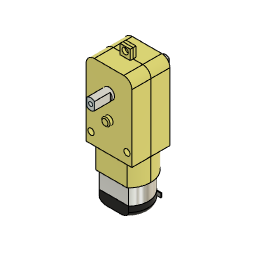
DC 3777 v3 (Autodesk Fusion 360 design; units mm, degrees)
Autodesk Fusion 360 part; units mm, degrees
sketch "main" plane through (0, 0, 0) normal (0, 1, 0) x (1, 0, 0)
  circle A0 centre (0, 0) radius 2.7
  line L0 (-11.2, -11.2) -> (11.2, -11.2)
  line L1 (11.2, -11.2) -> (11.2, 51)
  line L2 (11.2, 51) -> (-11.2, 51)
  line L3 (-11.2, 51) -> (-11.2, -11.2)
  line L4 (0, -11.2) -> (0, 51) construction
  line L5 (-2.5, -16) -> (2.5, -16)
  line L6 (2.5, -16) -> (2.5, -11.2)
  line L7 (2.5, -11.2) -> (-2.5, -11.2)
  line L8 (-2.5, -11.2) -> (-2.5, -16)
  circle A1 centre (0, -14) radius 1.5
  line L9 (-11.2, 25.8) -> (11.2, 25.8)
  line L10 (-1.85, 2.7) -> (1.85, 2.7)
  line L11 (1.85, 2.7) -> (1.85, -2.7)
  line L12 (1.85, -2.7) -> (-1.85, -2.7)
  line L13 (-1.85, -2.7) -> (-1.85, 2.7)
  line L14 (-1.85, 2.7) -> (1.85, -2.7) construction
  line L15 (1.85, 2.7) -> (-1.85, -2.7) construction
  circle A2 centre (8.8, 20.6) radius 1.5
  circle A3 centre (-8.8, 20.6) radius 1.5
  line L16 (8.8, 20.6) -> (-8.8, 20.6) construction
  circle A4 centre (0, 0) radius 0.975
  dimension "d1" = 5.4
  dimension "d2" = 22.4
  dimension "d3" = 62.2
  dimension "d4" = 11.2
  dimension "d5" = 5
  dimension "d7" = 3
  dimension "d8" = 2
  dimension "d10" = 3.7
  dimension "d11" = 5.4
  dimension "d21" = 3
  dimension "d22" = 8.8
  dimension "d23" = 3
  dimension "d24" = 8.8
  dimension "d25" = 31.8
  dimension "d52" = 37
  dimension "d61" = 1.95
  dimension "d62" = 4.8
  constraint coincident A0.centre A4.centre
  constraint horizontal L0
  constraint vertical L1
  constraint horizontal L2
  constraint vertical L3
  constraint midpoint L0 L4.start
  constraint midpoint L2 L4.end
  constraint coincident A0.centre L4
  constraint horizontal L5
  constraint vertical L6
  constraint horizontal L7
  constraint vertical L8
  constraint midpoint L0 L7
  constraint coincident L3 L9.start
  constraint coincident L1 L9.end
  constraint perpendicular L1 L9
  constraint perpendicular L10 L11
  constraint parallel L10 L12
  constraint parallel L11 L13
  constraint horizontal L10
  constraint coincident L14 A0.centre
  constraint coincident L15 A0.centre
  constraint coincident A2.centre L16.start
  constraint coincident A3.centre L16.end
  constraint horizontal L16
  measures "d1" diameter of A0
  measures "d2" distance of L0.start L0.end
  measures "d3" distance of L0.end L1.end
  measures "d4" distance of A0.centre L0
  measures "d5" distance of L5.start L5.end
  measures "d7" diameter of A1
  measures "d8" distance of L5 A1.centre
  measures "d10" distance of L11.end L12.end
  measures "d11" distance of L10.end L11.end
  measures "d21" diameter of A2
  measures "d22" distance of L4 A2.centre
  measures "d23" diameter of A3
  measures "d24" distance of L4 A3.centre
  measures "d25" distance of L0 A2.centre
  measures "d52" distance of L0 L9
  measures "d61" diameter of A4
  measures "d62" distance of L5.end L6.end
extrude "Extrude1" add sketch "main" along normal mid plane 18.6 contours A0 L10 L11 | A0 L11 L12 | A0 L10 L13 | A0 L12 L13 | L0 L1 L3 L7 L9 makes body 1
extrude "Extrude2" add sketch "main" along normal mid plane 2.8 contours L0 L5 L6 L7 L8 bodies 1
extrude "Extrude3" add sketch "main" along normal mid plane 21 separate body contours A0 L11 | A0 L11 L13 | A0 L13 | A4 makes body 2
extrude "Extrude4" add sketch "main" along normal mid plane 36.6 contours A0 L11 L13 bodies 2
fillet "Fillet1" radius 4 2 edges at (11.2, 0, 11.2) (-11.2, 0, 11.2) on bodies 1
sketch "bottom" plane through (0, 0, -25.8) normal (0, 0, -1) x (1, 0, 0)
  line L0 (-11.2, 9.3) -> (-11.2, -9.3)
  line L1 (-11.2, -9.3) -> (11.2, -9.3)
  line L2 (11.2, -9.3) -> (11.2, 9.3)
  line L3 (11.2, 9.3) -> (-11.2, 9.3)
  circle A0 centre (0, 0) radius 11.15
  line L4 (-11.2, 8.1) -> (11.2, 8.1)
  dimension "d26" = 22.3
  dimension "d29" = 1.2
  constraint coincident A0.centre origin
  constraint coincident L0 L4.start
  constraint coincident L2 L4.end
  constraint horizontal L4
  measures "d26" diameter of A0
  measures "d29" distance of L3 L4
extrude "Extrude5" add sketch "bottom" along normal blind 11 contours L1 A0 L4 bodies 1
sketch "more" plane through (0, 0, -36.8) normal (0, 0, -1) x (1, 0, 0)
  arc A0 (-7.6624, 8.1) -> (-6.1508, -9.3) centre (0, 0) ccw
  line L0 (-6.1508, -9.3) -> (6.1508, -9.3)
  arc A1 (6.1508, -9.3) -> (7.6624, 8.1) centre (0, 0) ccw
  line L1 (7.6624, 8.1) -> (-7.6624, 8.1)
  circle A2 centre (0, 0) radius 4.95
  arc A3 (-7.1689, 6.9) -> (-5.7786, -8.1) centre (0, 0) ccw
  line L2 (-5.7786, -8.1) -> (5.7786, -8.1)
  arc A4 (5.7786, -8.1) -> (7.1689, 6.9) centre (0, 0) ccw
  line L3 (7.1689, 6.9) -> (-7.1689, 6.9)
  line L4 (-5, 3.6) -> (5, 3.6)
  circle A5 centre (0, 0) radius 1
  dimension "d30" = 9.9
  dimension "d31" = 1.2
  dimension "d37" = 3.6
  dimension "d41" = 2
  constraint coincident A0.centre A1.centre
  constraint parallel L3 L4
  measures "d30" diameter of A2
  measures "d37" distance of A0.centre L4
  measures "d41" diameter of A5
extrude "Extrude6" add sketch "more" along normal blind 8.6 separate body contours A2 L4 | A2 L4 | A3 L2 A4 L3 | A5 makes body 3
extrude "Extrude7" add sketch "more" along normal blind 5.2 from surface at 8.6 separate body contours A2 L4 | A2 L4 | A3 L2 A4 L3 | A5 makes body 4
extrude "Extrude8" add sketch "more" along normal blind 2 from surface at 13.8 contours A2 L4 | A5 picked at (-0.0249, 2.7324) bodies 4
extrude "Extrude9" add sketch "more" along normal blind 2 from surface at 15.8 separate body contours A5 makes body 5
fillet "Fillet2" radius 1 1 edges at (-0.9323, 0.3616, -54.6) on bodies 5
sketch "nubber" plane through (0, -9.3, 0) normal (0, -1, 0) x (1, 0, 0)
  circle A0 centre (-8.8, -20.6) radius 1.5
  circle A1 centre (8.8, -20.6) radius 1.5
  arc A2 (-7.2, 11.2) -> (-11.2, 7.2) centre (-7.2, 7.2) ccw
  line L0 (-11.2, 7.2) -> (-11.2, -25.8)
  line L1 (-11.2, -25.8) -> (11.2, -25.8)
  line L2 (11.2, -25.8) -> (11.2, 7.2)
  arc A3 (11.2, 7.2) -> (7.2, 11.2) centre (7.2, 7.2) ccw
  line L3 (7.2, 11.2) -> (-7.2, 11.2)
  circle A4 centre (0, -11.25) radius 2
  circle A5 centre (0, 0) radius 2.7
  dimension "d46" = 4
  dimension "d47" = 11.25
  measures "d46" diameter of A4
  measures "d47" distance of A5.centre A4.centre
extrude "Extrude10" add sketch "nubber" along normal blind 2 contours A4 bodies 1
fillet "Fillet3" radius 0.5 1 edges at (-1.8647, -11.3, -11.9732) on bodies 1
fillet "Fillet4" radius 2.5 2 edges at (-9.9075, 0.9183, -50.6) (9.9075, 0.9183, -50.6) on bodies 4
split "Split1" by plane through (0, 0, 0) normal (0, 1, 0) bodies 1 makes body 6 at (0.0673, 9.3, -13.9506)
sketch "Sketch5" plane through (0, 8.1, 0) normal (0, 1, 0) x (-1, 0, 0)
  spline S0 degree 3 poles (5.7786, -48.1) (5.7786, -48.2998) (5.7259, -48.5338) (5.5453, -48.9398) (5.3678, -49.1736) (4.9234, -49.5927) (4.5434, -49.8136) (3.5837, -50.2134) (2.8684, -50.347) (1.4131, -50.4957) (0.6733, -50.514) (-0.6733, -50.514) (-1.4131, -50.4957) (-2.8684, -50.347) (-3.5837, -50.2134) (-4.5434, -49.8136) (-4.9234, -49.5927) (-5.3678, -49.1736) (-5.5453, -48.9398) (-5.7259, -48.5338) (-5.7786, -48.2998) (-5.7786, -48.1) knots 0.647214 0.647214 0.647214 0.647214 0.707165 0.707165 0.780538 0.780538 0.890431 0.890431 1.09243 1.09243 1.294429 1.294429 1.496428 1.496428 1.698427 1.698427 1.80832 1.80832 1.881693 1.881693 1.941643 1.941643 1.941643 1.941643
  line L0 (5.7786, -48.1) -> (5.7786, -45.4)
  line L1 (5.7786, -45.4) -> (-5.7786, -45.4)
  line L2 (-5.7786, -45.4) -> (-5.7786, -48.1)
  line L3 (-2, -47) -> (-8, -47)
  line L4 (-8, -47) -> (-8, -49)
  line L5 (-8, -49) -> (-2, -49)
  line L6 (-2, -49) -> (-2, -47)
  line L7 (2, -47) -> (8, -47)
  line L8 (8, -47) -> (8, -49)
  line L9 (8, -49) -> (2, -49)
  line L10 (2, -49) -> (2, -47)
  dimension "d53" = 6
  dimension "d54" = 2
  dimension "d55" = 2
  dimension "d56" = 6
  dimension "d57" = 2
  dimension "d58" = 4
  constraint horizontal L3
  constraint vertical L4
  constraint horizontal L5
  constraint vertical L6
  constraint horizontal L7
  constraint vertical L8
  constraint horizontal L9
  constraint vertical L10
  measures "d53" distance of L3.start L3.end
  measures "d54" distance of L3.start L5.end
  measures "d55" distance of origin L6
  measures "d56" distance of L7.start L7.end
  measures "d57" distance of L7.start L9.end
  measures "d58" distance of L6 L10
extrude "Extrude11" add sketch "Sketch5" along normal blind 0.4 separate body contours S0 L0 L7 L8 L9 | S0 L0 L7 L9 L10 | S0 L2 L3 L4 L5 | S0 L2 L3 L5 L6 makes body 7 at (-4, 8.1, -47.6667) makes body 8 at (4, 8.1, -48.3333)
sketch "Sketch6" plane through (0, -18.3, 0) normal (0, -1, 0) x (1, 0, 0)
  circle A0 centre (0, 0) radius 0.975
  arc A1 (-1.85, -1.9666) -> (1.85, -1.9666) centre (0, 0) ccw
  line L0 (1.85, -1.9666) -> (1.85, 1.9666)
  arc A2 (1.85, 1.9666) -> (-1.85, 1.9666) centre (0, 0) ccw
  line L1 (-1.85, 1.9666) -> (-1.85, -1.9666)
equation "d22 = ( 17.6 / 2 ) * 1 mm"
equation "d24 = ( 17.6 / 2 ) * 1 mm"
named bodies: "body A", "shaft", "metal bit", "cap", "pin thingy", "body B", "anode", "cathy"
